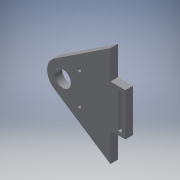
# Autodesk Inventor part: Mecanum wheel support
Saved by Autodesk Inventor 2018 (Build 220112000, 112)
## iProperties
Created: 2018-05-02
Part Number: Mecanum wheel support
Material: Generic
Document SubType Name: Modeling
Designer: Ajith Thomas
Density: 1 g/cm^3
Appearance: Default
Author: Ajith Thomas
Autodesk Inventor part; units mm, degrees
ref_plane "YZ Plane" through (0, 0, 0) normal (1, 0, 0) x (0, 1, 0)
ref_plane "XZ Plane" through (0, 0, 0) normal (0, 1, 0) x (-1, 0, 0)
ref_plane "XY Plane" through (0, 0, 0) normal (0, 0, 1) x (1, 0, 0)
sketch "Sketch1" plane through (0, 0, 0) normal (0, 0, 1) x (1, 0, 0)
  circle A0 centre (0, 0) radius 2 construction
  circle A1 centre (0, 0) radius 6.5 construction
  line L0 (0, 0) -> (38, 0) construction
  arc A2 (-6.8763, 10.4387) -> (-6.8763, -10.4387) centre (0, 0) ccw
  circle A3 centre (0, 0) radius 6.5
  line L1 (38, 0) -> (38, -40)
  line L2 (38, 0) -> (38, 40)
  line L3 (38, 40) -> (-6.8763, 10.4387)
  line L4 (38, -40) -> (-6.8763, -10.4387)
  point P0 (0, 0)
  dimension "d0" = 38
  dimension "d1" = 25
  dimension "d2" = 13
  dimension "d3" = 40
  dimension "d4" = 40
  constraints: 10 end point, 2 centre point, 2 coincident, 2 point on circle, 2 tangent, 2 vertical, 1 horizontal
  measures "d0" distance of L0.start L0.end
  measures "d1" diameter of A2
  measures "d2" diameter of A3
  measures "d3" distance of L0.end L1.end
  measures "d4" distance of L0.end L2.end
extrude "Extrusion1" add sketch "Sketch1" against normal blind 6
sketch "Sketch2" plane through (0, 0, -6) normal (0, 0, -1) x (-1, 0, 0)
  circle A0 centre (-13, -12.5) radius 1.5 projected
  circle A1 centre (-13, 12.5) radius 1.5 projected
  point P0 (0, 0)
extrude "Extrusion2" cut sketch "Sketch2" against normal blind 6
sketch "Sketch3" plane through (0, 0, -6) normal (0, 0, -1) x (-1, 0, 0)
  line L0 (-38, 40) -> (-38, -40) projected
  line L1 (-38, 40) -> (-38, -40) construction
  line L2 (-38, 0) -> (-63, 0) construction
  line L3 (-50, 0) -> (-50, -17)
  line L4 (-50, 0) -> (-50, 17)
  line L5 (-50, -17) -> (-38, -17)
  line L6 (-50, 17) -> (-38, 17)
  line L7 (-47.1, -14) -> (-47.1, 0)
  line L8 (-47.1, 14) -> (-47.1, 0)
  line L9 (-47.1, -14) -> (-44, -14)
  line L10 (-44, -14) -> (-44, 0)
  line L11 (-47.1, 14) -> (-44, 14)
  line L12 (-44, 14) -> (-44, 0)
  line L13 (-38, -17) -> (-38, 17)
  point P0 (0, 0)
  dimension "d9" = 25
  dimension "d10" = 17
  dimension "d11" = 12
  dimension "d12" = 14
  dimension "d13" = 2.9
  dimension "d14" = 6
  constraints: 24 end point, 4 point on line, 4 symmetric about line, 3 perpendicular, 2 horizontal, 1 collinear, 1 midpoint, 1 vertical
  measures "d9" distance of L2.start L2.end
  measures "d10" distance of L3.start L3.end
  measures "d11" distance between parallel lines of L0 L3
  measures "d12" distance of L7.start L7.end
  measures "d13" distance between parallel lines of L3 L7
  measures "d14" distance between parallel lines of L0 L12
extrude "Extrusion3" add sketch "Sketch3" against normal blind 6
body "Solid1"
